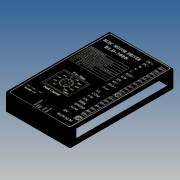
# Autodesk Inventor part: 800-20-MOTOR-CONTROLLER-BLD-300B-02
Saved by Autodesk Inventor 2018.2 (Build 222227000, 227)
## iProperties
Manager: feesmrt
Company: FRANCOR
Part Number: 800-20-MOTOR-CONTROLLER-BLD-300B-02
Material: Aluminium 6061
Document SubType Name: Modeling
Designer: feesmrt
Density: 2.7 g/cm^3
Appearance: Eloxiert - schwarz
Project: Rescue Robot
Cost Center: -
Engineer: feesmrt
Authority: feesmrt
Description: BLDC Motor Driver BLD-300B - Kühler
Stock Number: 800-20-MOTOR-CONTROLLER-BLD-300B-01
Author: feesmrt
Subject: Rescue Robot
Revision Number: 1
Title: BLDC Motor Driver BLD-300B - Deckel
Autodesk Inventor part; units mm, degrees
ref_plane "YZ Plane" through (0, 0, 0) normal (1, 0, 0) x (0, 1, 0)
ref_plane "XZ Plane" through (0, 0, 0) normal (0, 1, 0) x (-1, 0, 0)
ref_plane "XY Plane" through (0, 0, 0) normal (0, 0, 1) x (1, 0, 0)
sketch "Skizze1" plane through (0, 0, 0) normal (0, 0, 1) x (1, 0, 0)
  line L0 (-38.75, -63) -> (38.75, -63)
  line L1 (38.75, -63) -> (38.75, 63)
  line L2 (38.75, 63) -> (-38.75, 63)
  line L3 (-38.75, 63) -> (-38.75, -63)
  line L4 (-38.75, -63) -> (38.75, 63) construction
  line L5 (38.75, -63) -> (-38.75, 63) construction
  point P0 (0, 0)
  dimension "d23" = 77.5
  dimension "d24" = 126
  constraints: 12 end point, 2 midpoint, 2 parallel, 1 horizontal, 1 perpendicular
  measures "d23" distance of L1.end L2.end
  measures "d24" distance of L0.end L1.end
extrude "Grundkörper" add sketch "Skizze1" along normal blind 21
sketch "Skizze6" plane through (0, 0, 0) normal (0, 0, -1) x (-1, 0, 0)
  line L0 (-37.75, -62) -> (37.75, -62)
  line L1 (37.75, -62) -> (37.75, 62)
  line L2 (37.75, 62) -> (-37.75, 62)
  line L3 (-37.75, 62) -> (-37.75, -62)
  line L4 (-37.75, -62) -> (37.75, 62) construction
  line L5 (37.75, -62) -> (-37.75, 62) construction
  line L6 (-38.75, 63) -> (38.75, 63) projected
  line L7 (38.75, 63) -> (38.75, -63) projected
  point P0 (0, 0)
  dimension "d27" = 1
  dimension "d28" = 1
  constraints: 12 end point, 2 midpoint, 2 parallel, 1 horizontal, 1 perpendicular
  measures "d27" distance between parallel lines of L6 L2
  measures "d28" distance between parallel lines of L7 L1
extrude "Ausschnitt" cut sketch "Skizze6" against normal blind 20
sketch "Skizze8" plane through (38.75, -63, 0) normal (1, 0, 0) x (0, 0, -1)
  line L0 (0, 0) -> (-21, 0) construction
  line L1 (0, 0) -> (0, 126) construction
  line L2 (0, 126) -> (-21, 126) construction
  line L3 (-21, 0) -> (-21, 126) construction
  line L4 (-25.2, 63) -> (4.2, 63) construction
  line L5 (-6, 7.5) -> (-17, 7.5)
  line L6 (-17, 7.5) -> (-17, 118.5)
  line L7 (-17, 118.5) -> (-6, 118.5)
  line L8 (-6, 118.5) -> (-6, 7.5)
  line L9 (-6, 7.5) -> (-17, 118.5) construction
  line L10 (-17, 7.5) -> (-6, 118.5) construction
  point P0 (0, 63)
  point P1 (-11.5, 63)
  dimension "d32" = 7.5
  dimension "d33" = 6
  dimension "d34" = 4
  constraints: 12 end point, 2 midpoint, 2 parallel, 1 horizontal, 1 perpendicular, 1 point on line
  measures "d32" distance between parallel lines of L2 L7
  measures "d33" distance between parallel lines of L1 L8
  measures "d34" distance between parallel lines of L3 L6
extrude "Anschlüsse" cut sketch "Skizze8" against normal up to surface (1 mm away)
fillet "Rundung2" radius 1 5 edges at (38.75, 0, 21) (0, 63, 21) (0, -63, 21) (38.75, -63, 10.5) (38.75, 63, 10.5)
equation "\"d28\" = d27"
